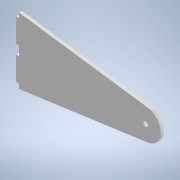
# Autodesk Inventor part: Base
Saved by Autodesk Inventor 2022 (Build 260153000, 153)
## iProperties
Created: 2022-02-08
Part Number: Base
Material: Generic
Document SubType Name: Modeling
Designer: katha
Density: 1 g/cm^3
Appearance: Default
Author: katha
Autodesk Inventor part; units mm, degrees
ref_plane "YZ Plane" through (0, 0, 0) normal (1, 0, 0) x (0, 1, 0)
ref_plane "XZ Plane" through (0, 0, 0) normal (0, 1, 0) x (-1, 0, 0)
ref_plane "XY Plane" through (0, 0, 0) normal (0, 0, 1) x (1, 0, 0)
sketch "Sketch2" plane through (0, 0, 0) normal (0, 0, 1) x (1, 0, 0)
  arc A0 (9.9386, -9.7664) -> (20.0614, -9.7664) centre (15, 0) ccw
  arc A1 (20.9272, -9.2665) -> (25.9886, -0.4999) centre (15, 0) ccw
  arc A2 (25.9886, 0.4999) -> (20.9272, 9.2665) centre (15, 0) ccw
  arc A3 (20.0614, 9.7664) -> (9.9386, 9.7664) centre (15, 0) ccw
  arc A4 (9.0728, 9.2665) -> (4.0114, 0.4999) centre (15, 0) ccw
  arc A5 (4.0114, -0.4999) -> (9.0728, -9.2665) centre (15, 0) ccw
  circle A6 centre (15, 0) radius 2.5
  arc A7 (0, -3) -> (12, -15) centre (12, -3) ccw
  circle A8 centre (15, 0) radius 16.1883
  line L0 (31.1883, 0) -> (-118.8117, 0) construction
  line L1 (-118.8117, 0) -> (-118.8117, 35)
  line L2 (17.2352, 16.0332) -> (-118.8117, 35)
  line L3 (-118.8117, 0) -> (-118.8117, -35)
  line L4 (17.2352, -16.0332) -> (-118.8117, -35)
  line L5 (-118.8117, -30) -> (-122.0117, -30)
  line L6 (-122.0117, -30) -> (-122.0117, -5)
  line L7 (-122.0117, -5) -> (-118.8117, -5)
  line L8 (-118.8117, 30) -> (-122.0117, 30)
  line L9 (-122.0117, 30) -> (-122.0117, 5)
  line L10 (-122.0117, 5) -> (-118.8117, 5)
  point P0 (0, 0)
  point P1 (5.2336, -12.9104)
  point P2 (2.0896, -9.7664)
extrude "Extrusion1" add sketch "Sketch2" along normal blind 3.2
body "Solid1"
